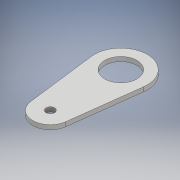
# Autodesk Inventor part: tipper_link_B_support
Saved by Autodesk Inventor 2017 (Build 210142000, 142)
## iProperties
Created: 2017-07-15
Part Number: tipper_link_B_support
Material: Generic
Document SubType Name: Modeling
Designer: Nic
Density: 1 g/cm^3
Appearance: Default
Author: Nic
Autodesk Inventor part; units mm, degrees
ref_plane "YZ Plane" through (0, 0, 0) normal (1, 0, 0) x (0, 1, 0)
ref_plane "XZ Plane" through (0, 0, 0) normal (0, 1, 0) x (-1, 0, 0)
ref_plane "XY Plane" through (0, 0, 0) normal (0, 0, 1) x (1, 0, 0)
sketch "Sketch1" plane through (0, 0, 0) normal (0, 0, 1) x (1, 0, 0)
  circle A0 centre (0, 0) radius 1.45
  line L0 (0, 0) -> (-32, 0) construction
  arc A1 (-6, 0) -> (5.9529, -0.75) centre (0, 0) ccw
  circle A2 centre (0, 24) radius 5.5
  arc A3 (8.9294, 22.875) -> (-8.9294, 22.875) centre (0, 24) ccw
  line L1 (8.9294, 22.875) -> (5.9529, -0.75)
  line L2 (-5.9529, -0.75) -> (-8.9294, 22.875)
  dimension "d0" = 2.9
  dimension "d61" = 6
  dimension "d63" = 24
  dimension "d69" = 9
  dimension "d72" = 11
  constraints: 6 end point, 5 point on circle, 4 centre point, 3 tangent, 2 coincident, 2 point on line, 1 concentric, 1 equal length, 1 vertical alignment
  measures "d0" diameter of A0
  measures "d61" radius of A1
  measures "d63" distance of point (0, 0) A2.centre
  measures "d69" radius of A3
  measures "d72" diameter of A2
extrude "Extrusion1" add sketch "Sketch1" along normal blind 1.5
body "Solid1"
